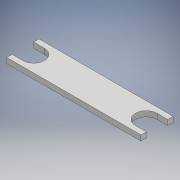
# Autodesk Inventor part: RescueKit-Slide
Saved by Autodesk Inventor 2018.3 (Build 223284000, 284)
## iProperties
Created: 2019-03-13
Part Number: RescueKit-Slide
Material: 一般
Document SubType Name: Modeling
Designer: shun2
Density: 1 g/cm^3
Appearance: 既定
Author: shun2
Autodesk Inventor part; units mm, degrees
ref_plane "YZ Plane" through (0, 0, 0) normal (1, 0, 0) x (0, 1, 0)
ref_plane "XZ Plane" through (0, 0, 0) normal (0, 1, 0) x (-1, 0, 0)
ref_plane "XY Plane" through (0, 0, 0) normal (0, 0, 1) x (1, 0, 0)
sketch "スケッチ1" plane through (0, 0, 0) normal (0, 0, 1) x (1, 0, 0)
  line L0 (0, 0) -> (125, 0)
  line L1 (125, 30) -> (0, 30)
  arc A0 (10, 5) -> (10, 25) centre (10, 15) ccw
  arc A1 (115, 25) -> (115, 5) centre (115, 15) ccw
  line L2 (10, 25) -> (0, 25)
  line L3 (10, 5) -> (0, 5)
  line L4 (115, 25) -> (125, 25)
  line L5 (115, 5) -> (125, 5)
  line L6 (0, 30) -> (0, 25)
  line L7 (0, 5) -> (0, 0)
  line L8 (125, 0) -> (125, 5)
  line L9 (125, 25) -> (125, 30)
  dimension "d0" = 125
  dimension "d1" = 30
  dimension "d2" = 20
  dimension "d3" = 20
  dimension "d7" = 125
  dimension "d9" = 5
  dimension "d12" = 10
  dimension "d15" = 115
  constraints: 20 end point, 6 perpendicular, 5 parallel, 4 point on circle, 4 point on line, 2 centre point, 2 tangent, 1 horizontal, 1 vertical
  measures "d0" distance of L1.end L1.start
  measures "d1" distance of L1.start L0.end
  measures "d2" diameter of A0
  measures "d3" diameter of A1
  measures "d7" distance between parallel lines of L8 L7
  measures "d9" distance of L3.end L0.start
  measures "d12" distance from line of A0.centre L7
  measures "d15" distance from line of L7 A1.centre
extrude "押し出し1" add sketch "スケッチ1" along normal blind 5
